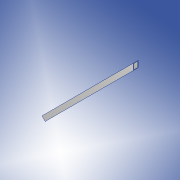
# Autodesk Inventor part: C004
Saved by Autodesk Inventor 2017 (Build 210142000, 142)
## iProperties
Created: 2017-06-13
Part Number: C004
Material: Aluminum 6061
Document SubType Name: Modeling
Designer: zallen
Density: 2.7 g/cm^3
Appearance: Aluminum - Flat
Mass: 151.351 g
Surface Area: 749.947 cm^2
Volume: 56.0559 cm^3
Author: zallen
Autodesk Inventor part; units mm, degrees
ref_plane "YZ Plane" through (0, 0, 0) normal (1, 0, 0) x (0, 1, 0)
ref_plane "XZ Plane" through (0, 0, 0) normal (0, 1, 0) x (-1, 0, 0)
ref_plane "XY Plane" through (0, 0, 0) normal (0, 0, 1) x (1, 0, 0)
sketch "Sketch2" plane through (0, 0, 0) normal (0, 0, 1) x (1, 0, 0)
  line L0 (0, 0) -> (377.5, 0) construction
  line L1 (377.5, 0) -> (377.5, 377.5) construction
  line L2 (0, 0) -> (377.5, 377.5) construction
  line L3 (-6.7175, 6.7175) -> (6.7175, -6.7175)
  line L4 (377.5, 390.935) -> (377.5, 364.065)
  line L5 (-6.7175, 6.7175) -> (377.5, 390.935)
  line L6 (6.7175, -6.7175) -> (377.5, 364.065)
  dimension "d4" = 377.5
  dimension "d5" = 377.5
  dimension "d6" = 19
  dimension "d7" = 90
  dimension "d13" = 45
  constraints: 14 end point, 2 midpoint, 1 horizontal, 1 perpendicular, 1 point on line
  measures "d4" distance of L0.start L0.end
  measures "d5" distance of L1.end L0.end
  measures "d6" distance of L3.start L3.end
  measures "d7" angle of L2 L3
  measures "d13" angle of L0 L6
extrude "Extrusion1" add sketch "Sketch2" along normal blind 19
sketch "Sketch3" plane through (6.7175, -6.7175, 19) normal (-0.7071, -0.7071, 0) x (-0.7071, 0.7071, 0)
  line L0 (19, 19) -> (0, 19) projected
  line L1 (0, 19) -> (0, 0) projected
  line L2 (19, 0) -> (0, 0) projected
  line L3 (19, 19) -> (19, 0) projected
  line L4 (17.5, 1.5) -> (1.5, 1.5)
  line L5 (1.5, 1.5) -> (1.5, 17.5)
  line L6 (1.5, 17.5) -> (17.5, 17.5)
  line L7 (17.5, 17.5) -> (17.5, 1.5)
  point P0 (9.5, 19)
  dimension "d14" = 1.5
  constraints: 8 end point, 3 other
  measures "d14" distance between parallel lines of L3 L7
extrude "Extrusion2" cut sketch "Sketch3" against normal through all contours L4 L5 L6 L7
body "Solid1"
